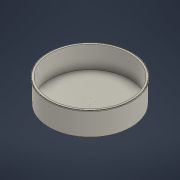
# Autodesk Inventor part: DomeFloor
Saved by Autodesk Inventor 2022 (Build 260153000, 153)
## iProperties
Created: 2021-05-07
Part Number: DomeFloor
Material: Generic
Document SubType Name: Modeling
Designer: Mick Veldhuis
Density: 1 g/cm^3
Appearance: Default
Author: Mick Veldhuis
Autodesk Inventor part; units mm, degrees
ref_plane "YZ Plane" through (0, 0, 0) normal (1, 0, 0) x (0, 1, 0)
ref_plane "XZ Plane" through (0, 0, 0) normal (0, 1, 0) x (-1, 0, 0)
sketch "Sketch1" plane through (0, 0, 0) normal (0, 1, 0) x (-1, 0, 0)
  circle A0 centre (0, 0) radius 3350
  dimension "d1" = 6700
  constraints: 1 centre point, 1 coincident
  measures "d1" diameter of A0
extrude "Extrusion1" add sketch "Sketch1" along normal blind 100
ref_plane "Work Plane3" through (0, 100, 0) normal (0, 1, 0) x (1, 0, 0)
sketch "Sketch5" plane through (0, 100, 0) normal (0, 1, 0) x (1, 0, 0)
  point P0 (180, -230)
  point P1 (-180, -230)
  point P2 (180, 230)
  point P3 (-180, 230)
hole "Hole1" at (180, 100, 230) at (-180, 100, 230) at (180, 100, -230) at (-180, 100, -230) direction (0, -1, 0) diameter 10.106 end through all thread size "M12x1.75" class "6H" standard "ISO Metric profile"
sketch "Sketch6" plane through (0, 100, 0) normal (0, 1, 0) x (1, 0, 0)
  circle A0 centre (0, 0) radius 2971.8
  circle A1 centre (0, 0) radius 3073.3
  circle A2 centre (0, 0) radius 3350 projected
  circle A3 centre (0, 0) radius 3350
  dimension "d19" = 5943.6
  dimension "d20" = 6146.6
  constraints: 3 centre point, 3 coincident
  measures "d19" diameter of A0
  measures "d20" diameter of A1
extrude "Extrusion5" cut sketch "Sketch6" against normal through all contours A2
extrude "Extrusion6" add sketch "Sketch6" along normal blind 1600 contours A1
ref_plane "Work Plane4" through (0, 1700, 0) normal (0, 1, 0) x (1, 0, 0)
sketch "Sketch7" plane through (0, 1700, 0) normal (0, 1, 0) x (1, 0, 0)
  circle A0 centre (0, 0) radius 3.124
  circle A1 centre (0, 0) radius 3124
  circle A2 centre (0, 0) radius 3100
  circle A3 centre (0, 0) radius 3073.3 projected
  circle A4 centre (0, 0) radius 2971.8
  circle A5 centre (0, 0) radius 3150
  constraints: 5 centre point, 5 coincident
extrude "Extrusion7" add sketch "Sketch7" along normal blind 60 contours A1 | A2 | A3 | A5
sketch "Sketch8" plane through (0, 1760, 0) normal (0, 1, 0) x (1, 0, 0)
  circle A0 centre (0, 0) radius 3124
  circle A1 centre (0, 0) radius 3100
  constraints: 2 centre point, 2 coincident
extrude "Extrusion8" cut sketch "Sketch8" against normal blind 40
body "Solid1"
